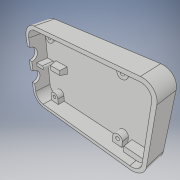
# Autodesk Inventor part: Case_Bottom
Saved by Autodesk Inventor 2019 (Build 230136000, 136)
## iProperties
Created: 2025-01-19
Part Number: Case_Bottom
Material: Générique
Document SubType Name: Modeling
Designer: Maxime
Density: 1 g/cm^3
Appearance: Par défaut
Author: Maxime
Autodesk Inventor part; units mm, degrees
ref_plane "XZ Plane" through (0, 0, 0) normal (0, 1, 0) x (-1, 0, 0)
ref_plane "XY Plane" through (0, 0, 0) normal (0, 0, 1) x (1, 0, 0)
sketch "Esquisse1" plane through (0, 0, 0) normal (0, 0, 1) x (1, 0, 0)
  line L0 (53.2, -33.2) -> (-53.2, -33.2)
  line L1 (-53.2, -33.2) -> (-53.2, 33.2)
  line L2 (-53.2, 33.2) -> (53.2, 33.2)
  line L3 (53.2, 33.2) -> (53.2, -33.2)
  line L4 (53.2, -33.2) -> (-53.2, 33.2) construction
  line L5 (-53.2, -33.2) -> (53.2, 33.2) construction
  point P0 (0, 0)
  dimension "d0" = 66.4
  dimension "d1" = 106.4
  constraints: 12 end point, 2 midpoint, 2 parallel, 1 horizontal, 1 perpendicular
  measures "d0" distance of L0.end L1.end
  measures "d1" distance between parallel lines of L3 L1
extrude "Extrusion1" add sketch "Esquisse1" along normal blind 16.95
shell "Coque1" thickness 3 removed faces 1 at (17.7333, 11.0667, 16.95)
ref_plane "PCBRestingPlane" through (-50.2, -30.2, 9) normal (0, 0, 1) x (1, 0, 0)
sketch "Esquisse2" plane through (-50.2, -30.2, 9) normal (0, 0, 1) x (1, 0, 0)
  line L0 (75.5, 5.2) -> (12.5, 5.2)
  line L1 (12.5, 5.2) -> (12.5, 54.2)
  line L2 (12.5, 54.2) -> (75.5, 54.2)
  line L3 (75.5, 54.2) -> (75.5, 5.2)
  line L4 (75.5, 5.2) -> (12.5, 54.2) construction
  line L5 (12.5, 5.2) -> (75.5, 54.2) construction
  line L6 (0, 0) -> (0, 60.4) projected
  circle A0 centre (12.5, 54.2) radius 4
  line L7 (8.5, 54.2) -> (8.5, 60.4)
  line L8 (0, 60.4) -> (100.4, 60.4) projected
  line L9 (16.5, 54.2) -> (16.5, 60.4)
  line L10 (16.5, 60.4) -> (8.5, 60.4)
  line L11 (50.2, 30.2) -> (44, 29.7)
  circle A1 centre (12.5, 5.2) radius 4
  line L12 (8.5, 5.2) -> (8.5, 0)
  line L13 (100.4, 0) -> (0, 0) projected
  line L14 (16.5, 5.2) -> (16.5, 0)
  line L15 (8.5, 0) -> (16.5, 0)
  dimension "d6" = 63
  dimension "d7" = 49
  dimension "d8" = 12.5
  dimension "d9" = 8
  dimension "d26" = 0.5
  dimension "d27" = 8
  constraints: 26 end point, 6 point on line, 4 parallel, 4 point on circle, 4 tangent, 3 horizontal, 2 centre point, 2 coincident, 2 midpoint, 2 vertical, 1 perpendicular
  measures "d6" distance of L1.end L2.end
  measures "d7" distance of L0.end L1.end
  measures "d8" distance between parallel lines of L6 L1
  measures "d9" diameter of A0
  measures "d26" vertical distance of L11.start L11.end
  measures "d27" diameter of A1
ref_plane "PCBMiddle" through (-6.2, -0.5, 9) normal (1, 0, 0) x (0, 1, 0)
extrude "Extrusion2" add sketch "Esquisse2" against normal up to next contours A1 L1 L0 | L14 L13 L12 A1 | L0 L1 A1 | A0 L1 L2 | L2 L1 A0 | A0 L7 L8 L9
mirror "Symétrie1" about plane through (-6.2, -0.5, 9) normal (1, 0, 0) of "Extrusion2"
ref_plane "Countersunk_Offset" through (0, 0, 3) normal (0, 0, -1) x (-1, 0, 0)
sketch "Esquisse3" plane through (0, 0, 3) normal (0, 0, -1) x (-1, 0, 0)
  point P0 (0, 0)
  point P1 (37.7, -25)
  point P2 (37.7, 24)
  point P3 (-25.3, 24)
  point P4 (-25.3, -25)
hole "Perçage1" at (-37.7, -25, 3) at (-37.7, 24, 3) at (25.3, 24, 3) at (25.3, -25, 3) direction (0, 0, 1) diameter 3.25 end through all start extended yes countersink diameter 6.2 countersink angle 90
sketch "Esquisse4" plane through (-53.2, -33.2, 0) normal (-1, 0, 0) x (0, 0, 1)
  line L0 (16.95, 3) -> (16.95, 63.4) projected
  circle A0 centre (16.95, 42.725) radius 5.6
  circle A1 centre (16.95, 23.675) radius 5.6
  line L1 (0, 33.2) -> (16.95, 33.2)
  dimension "d20" = 11.2
  dimension "d21" = 11.2
  dimension "d22" = 19.05
  dimension "d23" = 9.525
  constraints: 2 centre point, 2 end point, 2 point on line, 1 midpoint
  measures "d20" diameter of A0
  measures "d21" diameter of A1
  measures "d22" distance of A1.centre A0.centre
  measures "d23" distance from line of L1 A0.centre
extrude "Extrusion3" cut sketch "Esquisse4" against normal up to surface (3 mm away)
sketch "Esquisse5" plane through (50.2, -30.2, 3) normal (0, 0, 1) x (1, 0, 0)
  line L0 (-100.4, 0) -> (-100.4, 60.4) projected
  line L1 (-100.4, 31.65) -> (-92.4, 31.65)
  line L2 (-92.4, 31.65) -> (-92.4, 28.75)
  line L3 (-92.4, 28.75) -> (-100.4, 28.75)
  line L4 (-100.4, 28.75) -> (-100.4, 31.65)
  point P0 (-50.2, 30.2)
  point P1 (-100.4, 30.2)
  dimension "d28" = 8
  dimension "d29" = 2.9
  constraints: 8 end point, 2 midpoint, 2 parallel, 1 horizontal, 1 perpendicular, 1 point on line
  measures "d28" distance of L2.end L3.end
  measures "d29" distance of L1.end L2.end
extrude "Extrusion4" add sketch "Esquisse5" along normal blind 10
fillet "Congé1" radius 1.45 2 edges at (-42.2, -1.45, 8) (-42.2, 1.45, 8)
fillet "Congé2" radius 8 4 edges at (-50.2, 30.2, 9.975) (-50.2, -30.2, 9.975) (50.2, -30.2, 9.975) (50.2, 30.2, 9.975)
fillet "Congé2" radius 11 4 edges at (-53.2, 33.2, 8.475) (-53.2, -33.2, 8.475) (53.2, 33.2, 8.475) (53.2, -33.2, 8.475)
sketch "Esquisse6" plane through (-37.7, 24, 3) normal (0, 0, 1) x (1, 0, 0)
  line L0 (79.9, -54.2) -> (67, -54.2) projected
  line L1 (87.9, -1.8) -> (87.9, -46.2) projected
  line L2 (69.9, -54.2) -> (79.9, -54.2)
  line L3 (87.3162, -49.2) -> (69.9, -49.2)
  line L4 (69.9, -49.2) -> (69.9, -54.2)
  arc A0 (79.9, -54.2) -> (87.9, -46.2) centre (79.9, -46.2) ccw projected
  arc A1 (79.9, -54.2) -> (87.9, -46.2) centre (79.9, -46.2) ccw projected
  line L5 (87.9, -9.2) -> (86.9, -9.2)
  line L6 (86.9, -9.2) -> (86.9, -49.2)
  line L7 (86.9, -49.2) -> (87.9, -49.2)
  line L8 (87.9, -49.2) -> (87.9, -9.2)
  point P0 (37.7, -24)
  dimension "d36" = 5
  dimension "d37" = 18
  dimension "d40" = 1
  dimension "d41" = 40
  constraints: 14 end point, 3 parallel, 3 point on line, 2 horizontal, 2 point on circle, 1 perpendicular
  measures "d36" distance between parallel lines of L0 L3
  measures "d37" distance between parallel lines of L1 L4
  measures "d40" distance of L5.start L5.end
  measures "d41" distance of L5.end L6.end
extrude "Extrusion5" add sketch "Esquisse6" along normal blind 8
sketch "Esquisse7" plane through (-37.7, 24, 9) normal (0, 0, 1) x (1, 0, 0)
  line L0 (-1.5, -22) -> (8.5, -22)
  line L1 (8.5, -22) -> (8.5, -26)
  line L2 (8.5, -26) -> (-1.5, -26)
  line L3 (-1.5, -26) -> (-1.5, -22)
  line L4 (-1.5, -22) -> (8.5, -26) construction
  line L5 (8.5, -22) -> (-1.5, -26) construction
  line L6 (-12.5, -22.55) -> (-12.5, -1.8) projected
  line L7 (3.5, -24) -> (37.7, -24)
  dimension "d42" = 10
  dimension "d43" = 4
  dimension "d47" = 11
  constraints: 14 end point, 2 horizontal, 2 midpoint, 2 parallel, 1 perpendicular
  measures "d42" distance of L1.end L2.end
  measures "d43" distance of L0.end L1.end
  measures "d47" distance between parallel lines of L6 L3
extrude "Extrusion6" add sketch "Esquisse7" against normal up to surface (6 mm away) draft 10
equation "\"d27\" = d9"
equation "\"d21\" = d20"
equation "\"d23\" = 0.5 * d22"
equation "\"d32\" = 0.5 * d29"
